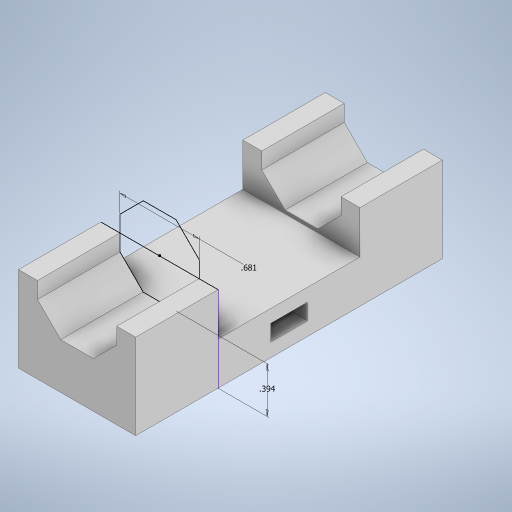
# Autodesk Inventor part: Gage Stand
Saved by Autodesk Inventor 2023 (Build 270158000, 158)
## iProperties
Created: 2024-04-04
Part Number: Gage Stand
Material: Generic
Document SubType Name: Modeling
Designer: Pobe Tran
Density: 1 g/cm^3
Appearance: Default
Author: Pobe Tran
Autodesk Inventor part; units mm, degrees
ref_plane "YZ Plane" through (0, 0, 0) normal (1, 0, 0) x (0, 1, 0)
ref_plane "XZ Plane" through (0, 0, 0) normal (0, 1, 0) x (-1, 0, 0)
ref_plane "XY Plane" through (0, 0, 0) normal (0, 0, 1) x (1, 0, 0)
sketch "Sketch1" plane through (0, 0, 0) normal (0, 0, 1) x (1, 0, 0)
  line L0 (8.65, 3.5829) -> (8.65, -3.5829)
  line L1 (8.65, -3.5829) -> (3.5829, -8.65)
  line L2 (3.5829, -8.65) -> (-3.5829, -8.65)
  line L3 (-3.5829, -8.65) -> (-8.65, -3.5829)
  line L4 (-8.65, -3.5829) -> (-8.65, 3.5829)
  line L5 (-8.65, 3.5829) -> (-3.5829, 8.65)
  line L6 (-3.5829, 8.65) -> (3.5829, 8.65)
  line L7 (3.5829, 8.65) -> (8.65, 3.5829)
  line L8 (-12.7904, 0) -> (12.7904, 0)
  line L9 (12.7904, 0) -> (12.7904, -18.65)
  line L10 (12.7904, -18.65) -> (-12.7904, -18.65)
  line L11 (-12.7904, -18.65) -> (-12.7904, 0)
  point P0 (0, 0)
  point P1 (0, 0)
  point P2 (0, 0)
  point P3 (-8.65, 0)
  point P4 (8.65, 0)
  dimension "d0" = 17.3
  dimension "d1" = 10
  constraints: 24 end point, 2 coincident, 2 parallel, 1 horizontal, 1 midpoint, 1 perpendicular, 1 vertical, 17 other
  measures "d0" distance between parallel lines of L0 L4
  measures "d1" distance between parallel lines of L10 L2
extrude "Extrusion1" add sketch "Sketch1" along normal blind 18 contours L8 L9 L10 L11 L4 L3 L2 L1 L0
sketch "Sketch2" plane through (0, 0, 0) normal (0, 0, -1) x (-1, 0, 0)
  line L0 (-12.7904, -18.65) -> (-12.7904, 0) projected
  line L1 (12.7904, 0) -> (12.7904, -18.65) projected
  line L2 (-12.7904, -18.65) -> (12.7904, -18.65)
  line L3 (12.7904, -18.65) -> (12.7904, -9.275)
  line L4 (12.7904, -9.325) -> (-12.7904, -9.325)
  line L5 (-12.7904, -9.325) -> (-12.7904, -18.65)
  point P0 (0, 0)
  point P1 (-12.7904, -9.325)
  constraints: 8 end point, 1 horizontal, 1 midpoint, 1 parallel, 1 perpendicular
extrude "Extrusion2" add sketch "Sketch2" along normal blind 31
extrude "Extrusion3" add sketch "Sketch1" against normal blind 18 from surface at -31 contours L8 L9 L10 L11 L4 L3 L2 L1 L0
sketch "Sketch3" plane through (12.7904, -18.65, 18) normal (1, 0, 0) x (0, 0, -1)
  line L0 (29.5, 6.5107) -> (37.5, 6.5107)
  line L1 (37.5, 6.5107) -> (37.5, 3.0107)
  line L2 (37.5, 3.0107) -> (29.5, 3.0107)
  line L3 (29.5, 3.0107) -> (29.5, 6.5107)
  line L4 (29.5, 6.5107) -> (37.5, 3.0107) construction
  line L5 (37.5, 6.5107) -> (29.5, 3.0107) construction
  line L6 (18, 9.325) -> (49, 9.325) projected
  point P0 (18, 18.65)
  point P1 (33.5, 4.7607)
  point P2 (33.5, 9.325)
  dimension "d8" = 3.5
  dimension "d9" = 8
  constraints: 12 end point, 3 midpoint, 2 parallel, 1 horizontal, 1 perpendicular, 1 vertical alignment
  measures "d8" distance of L0.end L1.end
  measures "d9" distance of L1.end L2.end
extrude "Extrusion4" cut sketch "Sketch3" against normal through all
body "Solid1"
